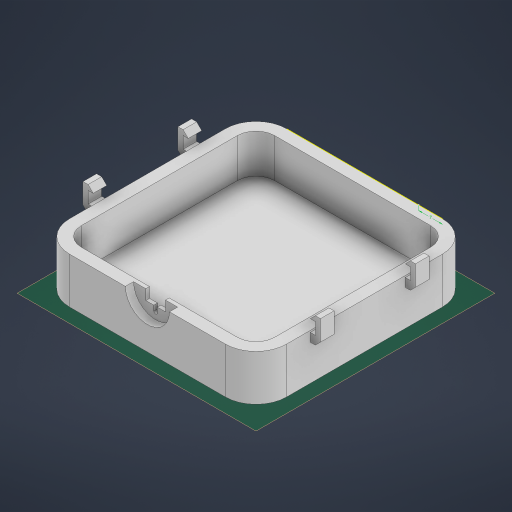
# Autodesk Inventor part: enclosure_i
Saved by Autodesk Inventor 2024.1 (Build 281209000, 209)
## iProperties
Created: 2023-07-19
Part Number: enclosure_i
Material: Generic
Document SubType Name: Modeling
Designer: LabTel_Admin
Density: 1 g/cm^3
Appearance: Default
Author: LabTel_Admin
Autodesk Inventor part; units mm, degrees
ref_plane "YZ Plane" through (0, 0, 0) normal (1, 0, 0) x (0, 1, 0)
ref_plane "XZ Plane" through (0, 0, 0) normal (0, 1, 0) x (-1, 0, 0)
ref_plane "XY Plane" through (0, 0, 0) normal (0, 0, 1) x (1, 0, 0)
sketch "Sketch1" plane through (0, 0, 0) normal (0, 1, 0) x (-1, 0, 0)
  line L0 (-23, -32) -> (23, -32)
  line L1 (32, -23) -> (32, 23)
  line L2 (23, 32) -> (-23, 32)
  line L3 (-32, 23) -> (-32, -23)
  line L4 (-32, -32) -> (32, 32) construction
  line L5 (32, -32) -> (-32, 32) construction
  arc A0 (32, 23) -> (23, 32) centre (23, 23) ccw
  arc A1 (23, -32) -> (32, -23) centre (23, -23) ccw
  arc A2 (-32, -23) -> (-23, -32) centre (-23, -23) ccw
  arc A3 (-23, 32) -> (-32, 23) centre (-23, 23) ccw
  line L6 (28.5, 23) -> (28.5, -23)
  arc A4 (23, -28.5) -> (28.5, -23) centre (23, -23) ccw
  line L7 (23, -28.5) -> (-23, -28.5)
  arc A5 (-28.5, -23) -> (-23, -28.5) centre (-23, -23) ccw
  line L8 (-28.5, -23) -> (-28.5, 23)
  arc A6 (-23, 28.5) -> (-28.5, 23) centre (-23, 23) ccw
  line L9 (-23, 28.5) -> (23, 28.5)
  arc A7 (28.5, 23) -> (23, 28.5) centre (23, 23) ccw
  point P0 (0, 0)
  point P1 (32, 0)
  point P2 (31.5, 26.5247)
  dimension "d0" = 64
  dimension "d1" = 64
  dimension "d3" = 9
  dimension "d4" = 9
  dimension "d5" = 3.5
  constraints: 20 end point, 16 point on circle, 8 centre point, 8 point on line, 8 tangent, 4 parallel, 3 midpoint, 2 equal radius, 2 perpendicular, 1 horizontal, 7 other
  measures "d0" distance of L5.end L4.end
  measures "d1" distance of L4.end L5.start
  measures "d3" radius of A0
  measures "d4" radius of A1
  measures "d5" distance between parallel lines of L1 L6
extrude "Extrusion1" add sketch "Sketch1" along normal blind 2 contours L6 A4 L7 A5 L8 A6 L9 A7
extrude "Extrusion2" add sketch "Sketch1" along normal blind 13.5
sketch "Sketch2" plane through (-23, 0, 32) normal (0, 0, 1) x (1, 0, 0)
  line L0 (0, 13.5) -> (46, 13.5) projected
  arc A0 (16.5, 13.5) -> (29.5, 13.5) centre (23, 13.5) ccw
  line L1 (16.5, 13.5) -> (29.5, 13.5)
  point P0 (23, 0)
  dimension "d10" = 13
  constraints: 2 end point, 2 point on circle, 2 point on line, 1 centre point, 1 collinear, 1 midpoint
  measures "d10" diameter of A0
extrude "Extrusion3" cut sketch "Sketch2" against normal blind 2.4
sketch "Sketch3" plane through (-23, 0, 29.6) normal (0, 0, 1) x (1, 0, 0)
  line L0 (25.9, 10.5) -> (20.1, 10.5)
  line L1 (20.1, 10.5) -> (20.1, 13.5)
  line L2 (25.9, 13.5) -> (25.9, 10.5)
  line L3 (16.5, 13.5) -> (29.5, 13.5) projected
  line L4 (25.9, 10.5) -> (23, 13.5) construction
  line L5 (20.1, 10.5) -> (25.9, 16.5) construction
  line L6 (20.1, 13.5) -> (25.9, 13.5)
  line L7 (23.5, 10.5) -> (23.5, 9)
  line L8 (23, 8.5) -> (23, 8.5)
  line L9 (22.5, 9) -> (22.5, 10.5)
  line L10 (23, 10.5) -> (23.5, 8.5) construction
  line L11 (23, 10.5) -> (22.5, 8.5) construction
  arc A0 (23, 8.5) -> (23.5, 9) centre (23, 9) ccw
  arc A1 (22.5, 9) -> (23, 8.5) centre (23, 9) ccw
  point P0 (23, 0)
  dimension "d13" = 6
  dimension "d15" = 1
  dimension "d17" = 0.5
  constraints: 22 end point, 8 point on line, 5 midpoint, 4 point on circle, 4 tangent, 2 centre point, 2 parallel, 1 concentric, 1 horizontal, 1 perpendicular
  measures "d13" distance of L5.end L0.start
  measures "d15" distance of L10.end L11.end
  measures "d17" radius of A0
extrude "Extrusion4" cut sketch "Sketch3" against normal blind 2
ref_plane "Work Plane1" through (0, -1, 0) normal (0, -1, 0) x (1, 0, 0)
sketch "Sketch5" plane through (0, -1, 0) normal (0, -1, 0) x (1, 0, 0)
  line L0 (-30.0692, 3.0119) -> (30.4708, 3.0119) construction
  line L1 (30.4708, 3.0119) -> (30.4708, -30.1194) construction
  line L2 (30.4708, -30.1194) -> (-30.0692, -30.1194) construction
  line L3 (-30.0692, -30.1194) -> (-30.0692, 3.0119) construction
  line L4 (-9.6136, -3.095) -> (-7.5909, 2.905)
  line L5 (-7.5909, 2.905) -> (-6.6088, 2.905)
  line L6 (-6.6088, 2.905) -> (-4.5861, -3.095)
  line L7 (-4.5861, -3.095) -> (-5.4272, -3.095)
  line L8 (-5.4272, -3.095) -> (-5.9718, -1.4176)
  line L9 (-5.9718, -1.4176) -> (-8.2619, -1.4176)
  line L10 (-8.2619, -1.4176) -> (-8.8065, -3.095)
  line L11 (-8.8065, -3.095) -> (-9.6136, -3.095)
  line L12 (-6.1906, -0.7368) -> (-7.1193, 2.0881)
  line L13 (-7.1193, 2.0881) -> (-8.0431, -0.7368)
  line L14 (-8.0431, -0.7368) -> (-6.1906, -0.7368)
  spline S0 degree 2 poles (-2.3446, -3.202) (-2.9961, -3.202) (-3.9102, -2.9297) (-4.3138, -2.7352) knots 0 0 0 1 2 2 2
  line L15 (-4.3138, -2.7352) -> (-4.3138, -1.7336)
  line L16 (-4.3138, -1.7336) -> (-4.2554, -1.7336)
  spline S1 degree 2 poles (-4.2554, -1.7336) (-3.8616, -2.1031) (-2.8648, -2.5116) (-2.4029, -2.5116) knots 0 0 0 1 2 2 2
  spline S2 degree 2 poles (-2.4029, -2.5116) (-1.7417, -2.5116) (-1.0658, -1.9621) (-1.0658, -1.5099) knots 0 0 0 1 2 2 2
  spline S3 degree 2 poles (-1.0658, -1.5099) (-1.0658, -1.1501) (-1.4208, -0.7028) (-1.8049, -0.591) knots 0 0 0 1 2 2 2
  spline S4 degree 2 poles (-1.8049, -0.591) (-2.082, -0.5132) (-2.5439, -0.4062) (-2.8892, -0.3187) knots 0 0 0 1 2 2 2
  spline S5 degree 2 poles (-2.8892, -0.3187) (-3.2003, -0.236) (-3.6914, 0.0119) (-3.8811, 0.2113) knots 0 0 0 1 2 2 2
  spline S6 degree 2 poles (-3.8811, 0.2113) (-4.0658, 0.4106) (-4.27, 0.9455) (-4.27, 1.2956) knots 0 0 0 1 2 2 2
  spline S7 degree 2 poles (-4.27, 1.2956) (-4.27, 2.0249) (-3.1323, 3.0119) (-2.2522, 3.0119) knots 0 0 0 1 2 2 2
  spline S8 degree 2 poles (-2.2522, 3.0119) (-1.7465, 3.0119) (-0.8519, 2.8126) (-0.4678, 2.623) knots 0 0 0 1 2 2 2
  line L17 (-0.4678, 2.623) -> (-0.4678, 1.67)
  line L18 (-0.4678, 1.67) -> (-0.5261, 1.67)
  spline S9 degree 2 poles (-0.5261, 1.67) (-0.813, 1.9325) (-1.7076, 2.3215) (-2.1987, 2.3215) knots 0 0 0 1 2 2 2
  spline S10 degree 2 poles (-2.1987, 2.3215) (-2.753, 2.3215) (-3.4386, 1.8012) (-3.4386, 1.3782) knots 0 0 0 1 2 2 2
  spline S11 degree 2 poles (-3.4386, 1.3782) (-3.4386, 0.999) (-3.035, 0.5468) (-2.6558, 0.4447) knots 0 0 0 1 2 2 2
  spline S12 degree 2 poles (-2.6558, 0.4447) (-2.4029, 0.3766) (-1.6687, 0.2016) (-1.4256, 0.1286) knots 0 0 0 1 2 2 2
  spline S13 degree 2 poles (-1.4256, 0.1286) (-0.8081, -0.061) (-0.2344, -0.8244) (-0.2344, -1.3835) knots 0 0 0 1 2 2 2
  spline S14 degree 2 poles (-0.2344, -1.3835) (-0.2344, -1.7385) (-0.5212, -2.4192) (-0.7789, -2.6574) knots 0 0 0 1 2 2 2
  spline S15 degree 2 poles (-0.7789, -2.6574) (-1.0658, -2.92) (-1.7952, -3.202) (-2.3446, -3.202) knots 0 0 0 1 2 2 2
  spline S16 degree 2 poles (2.6732, -3.2214) (2.1433, -3.2214) (1.3556, -2.9443) (1.0784, -2.6672) knots 0 0 0 1 2 2 2
  spline S17 degree 2 poles (1.0784, -2.6672) (0.7624, -2.356) (0.5047, -1.4808) (0.5047, -0.8389) knots 0 0 0 1 2 2 2
  line L19 (0.5047, -0.8389) -> (0.5047, 2.905)
  line L20 (0.5047, 2.905) -> (1.3021, 2.905)
  line L21 (1.3021, 2.905) -> (1.3021, -0.8389)
  spline S18 degree 2 poles (1.3021, -0.8389) (1.3021, -1.2571) (1.4091, -1.8211) (1.5598, -2.0496) knots 0 0 0 1 2 2 2
  spline S19 degree 2 poles (1.5598, -2.0496) (1.7202, -2.2928) (2.2745, -2.5407) (2.6732, -2.5407) knots 0 0 0 1 2 2 2
  spline S20 degree 2 poles (2.6732, -2.5407) (3.0476, -2.5407) (3.6311, -2.2928) (3.7916, -2.0496) knots 0 0 0 1 2 2 2
  spline S21 degree 2 poles (3.7916, -2.0496) (3.9423, -1.8211) (4.0493, -1.262) (4.0493, -0.8584) knots 0 0 0 1 2 2 2
  line L22 (4.0493, -0.8584) -> (4.0493, 2.905)
  line L23 (4.0493, 2.905) -> (4.8467, 2.905)
  line L24 (4.8467, 2.905) -> (4.8467, -0.8389)
  spline S22 degree 2 poles (4.8467, -0.8389) (4.8467, -1.4662) (4.5938, -2.3608) (4.2729, -2.6672) knots 0 0 0 1 2 2 2
  spline S23 degree 2 poles (4.2729, -2.6672) (3.986, -2.9492) (3.2275, -3.2214) (2.6732, -3.2214) knots 0 0 0 1 2 2 2
  spline S24 degree 2 poles (7.6619, -3.202) (7.0104, -3.202) (6.0963, -2.9297) (5.6927, -2.7352) knots 0 0 0 1 2 2 2
  line L25 (5.6927, -2.7352) -> (5.6927, -1.7336)
  line L26 (5.6927, -1.7336) -> (5.751, -1.7336)
  spline S25 degree 2 poles (5.751, -1.7336) (6.1449, -2.1031) (7.1416, -2.5116) (7.6036, -2.5116) knots 0 0 0 1 2 2 2
  spline S26 degree 2 poles (7.6036, -2.5116) (8.2648, -2.5116) (8.9407, -1.9621) (8.9407, -1.5099) knots 0 0 0 1 2 2 2
  spline S27 degree 2 poles (8.9407, -1.5099) (8.9407, -1.1501) (8.5857, -0.7028) (8.2016, -0.591) knots 0 0 0 1 2 2 2
  spline S28 degree 2 poles (8.2016, -0.591) (7.9245, -0.5132) (7.4625, -0.4062) (7.1173, -0.3187) knots 0 0 0 1 2 2 2
  spline S29 degree 2 poles (7.1173, -0.3187) (6.8061, -0.236) (6.3151, 0.0119) (6.1254, 0.2113) knots 0 0 0 1 2 2 2
  spline S30 degree 2 poles (6.1254, 0.2113) (5.9407, 0.4106) (5.7365, 0.9455) (5.7365, 1.2956) knots 0 0 0 1 2 2 2
  spline S31 degree 2 poles (5.7365, 1.2956) (5.7365, 2.0249) (6.8742, 3.0119) (7.7543, 3.0119) knots 0 0 0 1 2 2 2
  spline S32 degree 2 poles (7.7543, 3.0119) (8.26, 3.0119) (9.1546, 2.8126) (9.5387, 2.623) knots 0 0 0 1 2 2 2
  line L27 (9.5387, 2.623) -> (9.5387, 1.67)
  line L28 (9.5387, 1.67) -> (9.4804, 1.67)
  spline S33 degree 2 poles (9.4804, 1.67) (9.1935, 1.9325) (8.2989, 2.3215) (7.8078, 2.3215) knots 0 0 0 1 2 2 2
  spline S34 degree 2 poles (7.8078, 2.3215) (7.2535, 2.3215) (6.5679, 1.8012) (6.5679, 1.3782) knots 0 0 0 1 2 2 2
  spline S35 degree 2 poles (6.5679, 1.3782) (6.5679, 0.999) (6.9715, 0.5468) (7.3507, 0.4447) knots 0 0 0 1 2 2 2
  spline S36 degree 2 poles (7.3507, 0.4447) (7.6036, 0.3766) (8.3377, 0.2016) (8.5809, 0.1286) knots 0 0 0 1 2 2 2
  spline S37 degree 2 poles (8.5809, 0.1286) (9.1984, -0.061) (9.7721, -0.8244) (9.7721, -1.3835) knots 0 0 0 1 2 2 2
  spline S38 degree 2 poles (9.7721, -1.3835) (9.7721, -1.7385) (9.4852, -2.4192) (9.2275, -2.6574) knots 0 0 0 1 2 2 2
  spline S39 degree 2 poles (9.2275, -2.6574) (8.9407, -2.92) (8.2113, -3.202) (7.6619, -3.202) knots 0 0 0 1 2 2 2
  point P0 (0, 0)
  constraints: 2 other
extrude "Extrusion5" add sketch "Sketch5" against normal blind 1
sketch "Sketch6" plane through (-32, 0, -23) normal (-1, 0, 0) x (0, 0, 1)
  line L0 (0, 13.5) -> (46, 13.5) projected
  line L1 (39, 13.5) -> (35, 13.5)
  line L2 (35, 13.5) -> (35, 10.5)
  line L3 (35, 10.5) -> (39, 10.5)
  line L4 (39, 10.5) -> (39, 13.5)
  point P0 (23, 0)
  point P1 (39, 12)
  point P2 (35, 13.5)
  dimension "d23" = 4
  dimension "d24" = 7
  dimension "d25" = 3
  constraints: 8 end point, 2 parallel, 1 horizontal, 1 midpoint, 1 perpendicular, 1 point on line
  measures "d23" distance of L3.end L2.end
  measures "d24" horizontal distance of L0.end point (39, 12)
  measures "d25" distance of L1.end L2.end
extrude "Extrusion6" add sketch "Sketch6" along normal blind 3
sketch "Sketch7" plane through (0, 13.5, 0) normal (0, 1, 0) x (1, 0, 0)
  line L0 (-35, -16) -> (-35, -12) projected
  line L1 (-32, -12) -> (-35, -12) projected
  line L2 (-35, -16) -> (-33.5, -16)
  line L3 (-33.5, -16) -> (-33.5, -12)
  line L4 (-33.5, -12) -> (-35, -12)
  line L5 (-35, -12) -> (-35, -16)
  point P0 (0, 0)
  constraints: 8 end point, 2 parallel, 1 horizontal, 1 midpoint, 1 perpendicular
extrude "Extrusion7" add sketch "Sketch7" along normal blind 4.5
sketch "Sketch8" plane through (-33.5, 13.5, 16) normal (1, 0, 0) x (0, 0, -1)
  line L0 (0, -3) -> (0, 4.5) projected
  line L1 (4, -3) -> (4, 4.5) projected
  line L2 (0, 4.5) -> (4, 4.5)
  line L3 (4, 4.5) -> (4, 3)
  line L4 (4, 3) -> (0, 3)
  line L5 (0, 3) -> (0, 4.5)
  point P0 (16, -13.5)
  point P1 (0, 3)
  dimension "d30" = 1.5
  constraints: 8 end point, 2 parallel, 1 horizontal, 1 perpendicular, 1 point on line
  measures "d30" distance of L2.end L3.end
extrude "Extrusion8" add sketch "Sketch8" along normal blind 1.5
sketch "Sketch9" plane through (-32, 10.5, 16) normal (0, 0, 1) x (1, 0, 0)
  line L0 (0, 6) -> (0, 7.5) projected
  line L1 (0, 6) -> (-1.5, 7.5)
  line L2 (-3, 7.5) -> (0, 7.5) projected
  line L3 (-1.5, 3) -> (-1.5, 6) projected
  line L4 (-1.5, 6) -> (0, 6) projected
  line L5 (-1.5, 7.5) -> (0, 7.5)
  line L6 (0, 0) -> (-3, 0) projected
  line L7 (-1.5, 0) -> (-3, 1.5)
  line L8 (-3, 0) -> (-3, 7.5) projected
  line L9 (-1.5, 0) -> (-3, 0)
  line L10 (-3, 0) -> (-3, 1.5)
  line L11 (0, 6) -> (-0.9024, 6) construction
  point P0 (32, -10.5)
  point P1 (-0.4512, 6)
  dimension "d33" = 0
  dimension "d40" = 45
  constraints: 12 end point, 3 midpoint, 2 horizontal, 2 point on line, 1 collinear, 1 perpendicular
  measures "d33" distance from line of L1.end L3
  measures "d40" angle of L1 L0
extrude "Extrusion9" cut sketch "Sketch9" against normal blind 5
mirror "Mirror1" about plane through (0, 0, 0) normal (0, 0, 1) of "Extrusion9", "Extrusion6", "Extrusion7", "Extrusion8"
mirror "Mirror2" about plane through (0, 0, 0) normal (1, 0, 0) of "Extrusion6", "Extrusion7", "Extrusion8", "Extrusion9", "Mirror1"
sketch "Sketch10" plane through (23, 0, -32) normal (0, 0, -1) x (-1, 0, 0)
  line L0 (0, 13.5) -> (46, 13.5) projected
  line L1 (0, 2) -> (0, 13.5) projected
  point P0 (23, 0)
  point P1 (7, 13.5)
  dimension "d39" = 7
  constraints: 1 point on line
  measures "d39" distance from line of L1 point (7, 13.5)
sketch "Sketch11" plane through (0, 13.5, 0) normal (0, 1, 0) x (1, 0, 0)
  line L0 (-32, -16) -> (-33.5, -16) projected
  line L1 (-32, -16) -> (-32, -12) projected
  line L2 (-33.5, -16) -> (-32, -16)
  line L3 (-32, -16) -> (-32, -12)
  line L4 (-32, -12) -> (-33.5, -12)
  line L5 (-33.5, -12) -> (-33.5, -16)
  point P0 (0, 0)
  constraints: 8 end point, 2 parallel, 1 horizontal, 1 perpendicular
extrude "Extrusion10" cut sketch "Sketch11" against normal blind 0.5
mirror "Mirror3" about plane through (0, 0, 0) normal (0, 0, 1) of "Extrusion10"
mirror "Mirror4" about plane through (0, 0, 0) normal (1, 0, 0) of "Extrusion10", "Mirror3"
body "Solid1"
